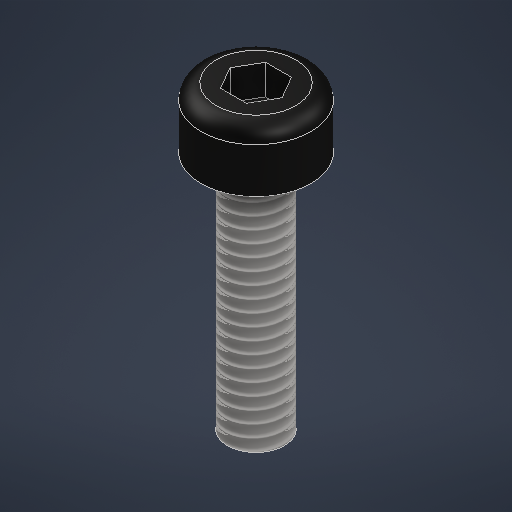
# Autodesk Inventor part: M2x16
Saved by Autodesk Inventor 2025.1 (Build 291241000, 241)
## iProperties
Created: 2024-10-26
Part Number: M2x16
Material: Generic
Document SubType Name: Modeling
Designer: jerem
Density: 1 g/cm^3
Appearance: Default
Author: jerem
Autodesk Inventor part; units mm, degrees
ref_plane "YZ Plane" through (0, 0, 0) normal (1, 0, 0) x (0, 1, 0)
ref_plane "XZ Plane" through (0, 0, 0) normal (0, 1, 0) x (-1, 0, 0)
ref_plane "XY Plane" through (0, 0, 0) normal (0, 0, 1) x (1, 0, 0)
sketch "Sketch1" plane through (0, 0, 0) normal (0, 1, 0) x (-1, 0, 0)
  circle A0 centre (0, 0) radius 0.95
  circle A1 centre (0, 0) radius 1.825
  line L0 (0.433, -0.75) -> (-0.433, -0.75)
  line L1 (-0.433, -0.75) -> (-0.866, 0)
  line L2 (-0.866, 0) -> (-0.433, 0.75)
  line L3 (-0.433, 0.75) -> (0.433, 0.75)
  line L4 (0.433, 0.75) -> (0.866, 0)
  line L5 (0.866, 0) -> (0.433, -0.75)
  dimension "d0" = 1.9
  dimension "d1" = 3.65
  dimension "d8" = 1.5
  constraints: 12 end point, 3 coincident, 2 centre point, 1 horizontal, 13 other
  measures "d0" diameter of A0
  measures "d1" diameter of A1
  measures "d8" distance between parallel lines of L3 L0
extrude "Extrusion1" add sketch "Sketch1" along normal blind 2 contours A0 | A1 | L0 L1 L2 L3 L4 L5
extrude "Extrusion2" add sketch "Sketch1" against normal blind 8 contours A0 | L0 L1 L2 L3 L4 L5
extrude "Extrusion3" cut sketch "Sketch1" against normal blind 1 from surface at 2 contours L0 L1 L2 L3 L4 L5
fillet "Fillet1" radius 0.5 1 edges at (1.825, 2, 0)
thread "Thread2" size "M2x0.4" class "6g" standard "ANSI Metric M Profile" full length
equation "\"d4\" = length"
equation "\"length\" = 8"
body "Solid1"
